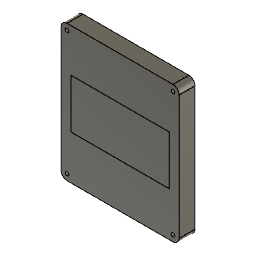
Back-display-o (Autodesk Fusion 360 design; units mm, degrees)
part number: 2026-02-05-20-27-14-774
Autodesk Fusion 360 part; units mm, degrees
sketch "Sketch1" plane through (0, 0, 0) normal (0, 1, 0) x (1, 0, 0)
  line L0 (33.4925, -50) -> (-62.7075, -50)
  line L1 (-62.7075, -50) -> (-62.7075, 61)
  line L2 (-62.7075, 61) -> (33.4925, 61)
  line L3 (33.4925, 61) -> (33.4925, -50)
  circle A0 centre (28.4925, -45) radius 1.5
  circle A1 centre (-57.7075, -45) radius 1.5
  circle A2 centre (-57.7075, 56) radius 1.5
  circle A3 centre (28.4925, 56) radius 1.5
  line L4 (25.4925, -14.9706) -> (-54.5075, -14.9706)
  line L5 (-54.5075, -14.9706) -> (-54.5075, 25.0294)
  line L6 (-54.5075, 25.0294) -> (25.4925, 25.0294)
  line L7 (25.4925, 25.0294) -> (25.4925, -14.9706)
  dimension "d1" = 96.2
  dimension "d2" = 111
  dimension "d3" = 3
  dimension "d4" = 5
  dimension "d5" = 5
  dimension "d6" = 3
  dimension "d7" = 5
  dimension "d8" = 5
  dimension "d9" = 3
  dimension "d10" = 5
  dimension "d11" = 5
  dimension "d12" = 3
  dimension "d13" = 5
  dimension "d14" = 5
  dimension "d15" = 40
  dimension "d16" = 80
  dimension "d21" = 8
  dimension "d22" = 35.0294
  constraint horizontal L0
  constraint vertical L1
  constraint horizontal L2
  constraint vertical L3
  constraint horizontal L4
  constraint vertical L5
  constraint horizontal L6
  constraint vertical L7
  measures "d1" distance of L1 L3
  measures "d2" distance of L0 L2
  measures "d3" diameter of A0
  measures "d4" distance of L3 A0.centre
  measures "d5" distance of L0 A0.centre
  measures "d6" diameter of A1
  measures "d7" distance of L1 A1.centre
  measures "d8" distance of L0 A1.centre
  measures "d9" diameter of A2
  measures "d10" distance of L1 A2.centre
  measures "d11" distance of L2 A2.centre
  measures "d12" diameter of A3
  measures "d13" distance of L2 A3.centre
  measures "d14" distance of L3 A3.centre
  measures "d15" distance of L4 L6
  measures "d16" distance of L5 L7
  measures "d21" distance of L3 L7
  measures "d22" distance of L0 L4
extrude "Extrude1" add sketch "Sketch1" along normal blind 13 makes body 1
extrude "Extrude2" add sketch "Sketch1" along normal blind 4 separate body contours L4 L5 L6 L7 makes body 2
sketch "Sketch4" plane through (0, 13, 0) normal (0, 1, 0) x (-1, 0, 0)
  circle A0 centre (57.7075, 45) radius 1.5
  circle A1 centre (57.7075, -56) radius 1.5
  circle A2 centre (-28.4925, -56) radius 1.5
  circle A3 centre (-28.4925, 45) radius 1.5
  line L0 (54.5075, -25.0294) -> (-25.4925, -25.0294)
  line L1 (-25.4925, -25.0294) -> (-25.4925, 14.9706)
  line L2 (-25.4925, 14.9706) -> (54.5075, 14.9706)
  line L3 (54.5075, 14.9706) -> (54.5075, -25.0294)
  line L4 (-33.4925, -61) -> (62.7075, -61)
  line L5 (62.7075, -61) -> (62.7075, 50)
  line L6 (62.7075, 50) -> (-33.4925, 50)
  line L7 (-33.4925, 50) -> (-33.4925, -61)
  line L8 (54.5075, 14.9706) -> (6.8436, 14.9706)
  line L9 (6.8436, 14.9706) -> (6.8436, 37.4505)
  line L10 (6.8436, 37.4505) -> (54.5075, 37.4505)
  line L11 (54.5075, 37.4505) -> (54.5075, 14.9706)
  dimension "d35" = 22.4799
  dimension "d36" = 47.6638
  constraint horizontal L8
  constraint vertical L9
  constraint horizontal L10
  constraint vertical L11
  constraint coincident L2.end L3.start
  measures "d35" distance of L8 L10
  measures "d36" distance of L9 L11
extrude "Extrude4" cut sketch "Sketch4" against normal blind 9 contours L2 L8 L9 L10 L11 bodies 1
fillet "Fillet1" radius 5 1 edges at (-62.7075, 6.5, 50) on bodies 1
fillet "Fillet2" radius 5 1 edges at (33.4925, 6.5, 50) on bodies 1
fillet "Fillet3" radius 5 1 edges at (33.4925, 6.5, -61) on bodies 1
fillet "Fillet4" radius 5 1 edges at (-62.7075, 6.5, -61) on bodies 1
